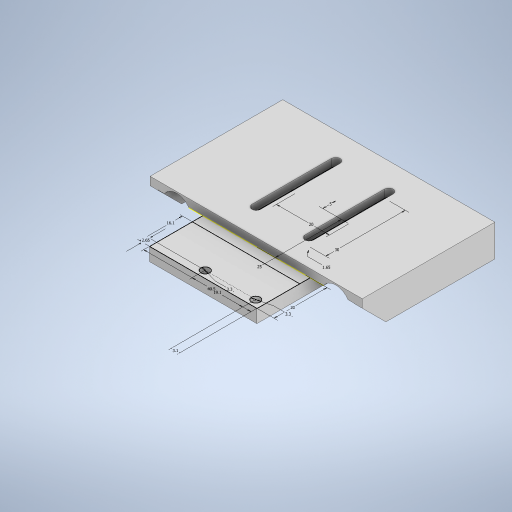
# Autodesk Inventor part: Soporte Y
Saved by Autodesk Inventor 2024 (Build 280153000, 153)
## iProperties
Created: 2024-06-03
Part Number: Soporte Y
Material: Generic
Document SubType Name: Modeling
Designer: juanp
Density: 1 g/cm^3
Appearance: Default
Author: juanp
Autodesk Inventor part; units mm, degrees
ref_plane "YZ Plane" through (0, 0, 0) normal (1, 0, 0) x (0, 1, 0)
ref_plane "XZ Plane" through (0, 0, 0) normal (0, 1, 0) x (-1, 0, 0)
ref_plane "XY Plane" through (0, 0, 0) normal (0, 0, 1) x (1, 0, 0)
sketch "Sketch1" plane through (0, 0, 0) normal (0, 0, 1) x (1, 0, 0)
  line L0 (40, -6) -> (-40, -6)
  line L1 (-40, -6) -> (-40, 6)
  line L2 (-40, 6) -> (40, 6)
  line L3 (40, 6) -> (40, -6)
  line L4 (40, -6) -> (-40, 6) construction
  line L5 (-40, -6) -> (40, 6) construction
  line L6 (-30, 0) -> (30, 0) construction
  circle A0 centre (-30, 0) radius 2.65
  circle A1 centre (30, 0) radius 2.65
  circle A2 centre (-30, 0) radius 5.5
  circle A3 centre (30, 0) radius 5.5
  line L7 (-40, 3) -> (40, 3)
  line L8 (-37, 6) -> (-37, -6)
  line L9 (37, 6) -> (37, -6)
  point P0 (0, 0)
  point P1 (-37, 3)
  point P2 (-34.6098, 3)
  point P3 (-25.3902, 3)
  point P4 (25.3902, 3)
  point P5 (34.6098, 3)
  point P6 (37, 3)
  dimension "d0" = 80
  dimension "d1" = 12
  dimension "d2" = 60
  dimension "d3" = 5.3
  dimension "d4" = 5.3
  dimension "d5" = 11
  dimension "d6" = 11
  dimension "d7" = 3
  dimension "d8" = 3
  dimension "d9" = 3
  constraints: 20 end point, 6 point on line, 4 centre point, 4 coincident, 4 perpendicular, 3 midpoint, 2 horizontal, 2 parallel
  measures "d0" distance of L1.end L2.end
  measures "d1" distance of L2.end L0.start
  measures "d2" distance of L6.start L6.end
  measures "d3" diameter of A0
  measures "d4" diameter of A1
  measures "d5" diameter of A2
  measures "d6" diameter of A3
  measures "d7" distance between parallel lines of L2 L7
  measures "d8" distance between parallel lines of L1 L8
  measures "d9" distance between parallel lines of L3 L9
extrude "Extrusion1" add sketch "Sketch1" along normal blind 3
extrude "Extrusion2" add sketch "Sketch1" along normal blind 50 contours L0 L9 L7 L3 | L7 L9 L2 L3 | L0 L1 L7 L8 | L7 A3 A2 L8 L2 L9 | L7 L1 L2 L8
chamfer "Chamfer1" distance 8.9 angle 45 2 edges at (-38.5, -6, 50) (38.5, -6, 50)
sketch "Sketch2" plane through (-25.3902, 3, 3) normal (0, -1, 0) x (1, 0, 0)
  line L0 (0, 47) -> (50.7805, 47) projected
  line L1 (25.3902, 47) -> (25.3902, 22) construction
  line L2 (35.3902, 22) -> (15.3902, 22) construction
  line L3 (35.3902, 7) -> (35.3902, 37) construction
  line L4 (37.0402, 7) -> (37.0402, 37)
  line L5 (33.7402, 37) -> (33.7402, 7)
  arc A0 (33.7402, 7) -> (37.0402, 7) centre (35.3902, 7) ccw
  arc A1 (37.0402, 37) -> (33.7402, 37) centre (35.3902, 37) ccw
  line L6 (15.3902, 7) -> (15.3902, 37) construction
  line L7 (17.0402, 7) -> (17.0402, 37)
  line L8 (13.7402, 37) -> (13.7402, 7)
  arc A2 (13.7402, 7) -> (17.0402, 7) centre (15.3902, 7) ccw
  arc A3 (17.0402, 37) -> (13.7402, 37) centre (15.3902, 37) ccw
  circle A4 centre (35.3902, 22) radius 1.65
  circle A5 centre (15.3902, 22) radius 1.65
  line L9 (45.6402, 67) -> (5.1402, 67)
  line L10 (5.1402, 67) -> (5.1402, 17)
  line L11 (5.1402, 17) -> (45.6402, 17)
  line L12 (45.6402, 17) -> (45.6402, 67)
  circle A6 centre (23.4402, 64.35) radius 1.65
  line L13 (42.5402, 64.35) -> (23.4402, 64.35) construction
  line L14 (45.6402, 50.9) -> (45.6402, 67)
  line L15 (5.1402, 50.9) -> (45.6402, 50.9)
  line L16 (5.1402, 67) -> (5.1402, 50.9)
  line L17 (45.6402, 67) -> (5.1402, 67)
  circle A7 centre (42.5402, 64.35) radius 1.65
  line L18 (25.3902, 22) -> (25.3902, 17)
  point P0 (25.3902, -3)
  dimension "d17" = 20
  dimension "d18" = 1.65
  dimension "d19" = 30
  dimension "d20" = 25
  dimension "d23" = 5
  dimension "d24" = 20
  dimension "d36" = 40.5
  dimension "d37" = 16.1
  dimension "d38" = 19.1
  dimension "d39" = 3.3
  dimension "d40" = 3.3
  dimension "d41" = 2.65
  dimension "d42" = 3.1
  constraints: 40 end point, 8 centre point, 8 parallel, 8 point on circle, 8 tangent, 5 midpoint, 4 coincident, 3 equal radius, 3 horizontal, 3 perpendicular, 2 vertical, 1 point on line
  measures "d17" distance of L2.start L2.end
  measures "d18" radius of A1
  measures "d19" distance of L3.start L3.end
  measures "d20" distance of L1.start L1.end
  measures "d23" distance from line of L11 A4.centre
  measures "d24" distance between parallel lines of L9 L0
  measures "d36" distance of L9.end L14.end
  measures "d37" distance of L9.end L15.start
  measures "d38" distance of L13.start L13.end
  measures "d39" diameter of A7
  measures "d40" diameter of A6
  measures "d41" distance between parallel lines of L13 L17
  measures "d42" distance from line of L13.start L14
extrude "Extrusion3" cut sketch "Sketch2" against normal through all contours L11 L7 A2 L8 | L8 A5 L7 L11 | L11 L5 A4 L4 | L4 A0 L5 L11 | L8 A3 L7 A5 | A5 | A4 L5 A1 L4 | A4
extrude "Extrusion4" add sketch "Sketch2" along normal blind 5 separate body contours L10 L15 L12 L0 | L0 L12 L11 L4 A1 L5 L7 A3 L8 L10 | L10 L9 L12 L15 | L8 A5 L7 L11 | L11 L5 A4 L4 | L8 A3 L7 A5 | A4 L5 A1 L4 | A6 | A7
extrude "Extrusion5" cut sketch "Sketch2" along normal through all contours A6 | A7 bodies 1 2
body "Solid1"
body "Solid2"
